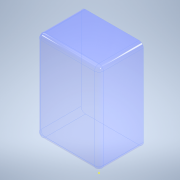
# Autodesk Inventor part: box
Saved by Autodesk Inventor 2022 (Build 260153000, 153)
## iProperties
Created: 2022-08-22
Part Number: box
Material: Glass
Document SubType Name: Modeling
Designer: Sachin
Density: 2.18 g/cm^3
Appearance: Clear - Blue
Author: Sachin
Autodesk Inventor part; units mm, degrees
ref_plane "YZ Plane" through (0, 0, 0) normal (1, 0, 0) x (0, 1, 0)
ref_plane "XZ Plane" through (0, 0, 0) normal (0, 1, 0) x (-1, 0, 0)
ref_plane "XY Plane" through (0, 0, 0) normal (0, 0, 1) x (1, 0, 0)
sketch "Sketch1" plane through (0, 0, 0) normal (0, 0, 1) x (1, 0, 0)
  line L0 (0, 0) -> (-70, 0)
  line L1 (-70, 0) -> (-70, 101.6)
  line L2 (-70, 101.6) -> (0, 101.6)
  line L3 (0, 101.6) -> (0, 0)
  dimension "d0" = 70
  dimension "d1" = 101.6
  constraints: 8 end point, 2 parallel, 1 horizontal, 1 perpendicular
  measures "d0" distance of L1.end L2.end
  measures "d1" distance of L0.end L1.end
extrude "Extrusion1" add sketch "Sketch1" along normal blind 50
fillet "Fillet1" radius 5 8 edges at (-70, 0, 25) (0, 0, 25) (-70, 101.6, 25) (0, 101.6, 25) (-70, 50.8, 50) (-35, 101.6, 50) (0, 50.8, 50) (-35, 0, 50)
sketch "Sketch2" plane through (0, 0, 50) normal (0, 0, 1) x (1, 0, 0)
  point P0 (0, 0)
body "Solid1"
